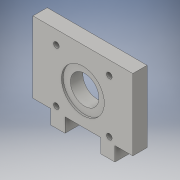
# Autodesk Inventor part: Motor Bracket
Saved by Autodesk Inventor 2016 (Build 200138000, 138)
## iProperties
Created: 2016-04-25
Part Number: Motor Bracket
Material: Generic
Document SubType Name: Modeling
Designer: rubenjm
Density: 1 g/cm^3
Appearance: Default
Author: rubenjm
Autodesk Inventor part; units mm, degrees
ref_plane "YZ Plane" through (0, 0, 0) normal (1, 0, 0) x (0, 1, 0)
ref_plane "XZ Plane" through (0, 0, 0) normal (0, 1, 0) x (-1, 0, 0)
ref_plane "XY Plane" through (0, 0, 0) normal (0, 0, 1) x (1, 0, 0)
sketch "Sketch1" plane through (0, 0, 0) normal (0, 0, 1) x (1, 0, 0)
  line L0 (0, 0) -> (15.875, 0)
  line L1 (88.9, 0) -> (88.9, 63.5)
  line L2 (88.9, 63.5) -> (0, 63.5)
  line L3 (0, 63.5) -> (0, 0)
  line L4 (44.45, 0) -> (60.325, 0) construction
  line L5 (44.45, 0) -> (60.325, 0) construction
  line L6 (73.025, 0) -> (73.025, -12.7)
  line L7 (73.025, -12.7) -> (60.325, -12.7)
  line L8 (60.325, -12.7) -> (60.325, 0)
  line L9 (73.025, 0) -> (88.9, 0)
  line L10 (44.45, 0) -> (44.45, 63.5) construction
  line L11 (44.45, 0) -> (28.575, 0) construction
  line L12 (44.45, 0) -> (28.575, 0) construction
  line L13 (15.875, 0) -> (15.875, -12.7)
  line L14 (15.875, -12.7) -> (28.575, -12.7)
  line L15 (28.575, -12.7) -> (28.575, 0)
  line L16 (28.575, 0) -> (60.325, 0)
  dimension "d10" = 88.9
  dimension "d11" = 63.5
  dimension "d12" = 15.875
  dimension "d13" = 0
  dimension "d14" = 12.7
  dimension "d15" = 12.7
  constraints: 34 end point, 5 parallel, 5 symmetric about line, 4 collinear, 4 horizontal, 3 perpendicular, 1 midpoint
  measures "d10" distance of L2.end L1.end
  measures "d11" distance of L1.end L1.start
  measures "d12" distance of L4.start L4.end
  measures "d13" distance between parallel lines of L4 L5
  measures "d14" distance of L6.end L7.end
  measures "d15" distance of L6.start L6.end
extrude "Extrusion1" add sketch "Sketch1" along normal blind 12.7
sketch "Sketch2" plane through (0, 0, 12.7) normal (0, 0, 1) x (1, 0, 0)
  line L0 (72.65, -0.26) -> (16.25, -0.26) construction
  line L1 (16.25, -0.26) -> (16.25, 56.14) construction
  line L2 (16.25, 56.14) -> (72.65, 56.14) construction
  line L3 (72.65, 56.14) -> (72.65, -0.26) construction
  line L4 (16.25, -0.26) -> (72.65, 56.14) construction
  line L5 (68.02, 4.37) -> (20.88, 4.37) construction
  line L6 (20.88, 4.37) -> (20.88, 51.51) construction
  line L7 (20.88, 51.51) -> (68.02, 51.51) construction
  line L8 (68.02, 51.51) -> (68.02, 4.37) construction
  line L9 (68.02, 4.37) -> (20.88, 51.51) construction
  line L10 (20.88, 4.37) -> (68.02, 51.51) construction
  circle A0 centre (20.8494, 4.3394) radius 2.5
  circle A1 centre (20.88, 51.51) radius 2.5
  circle A2 centre (68.02, 51.51) radius 2.5
  circle A3 centre (68.02, 4.37) radius 2.5
  line L11 (28.575, 0) -> (60.325, 0) construction
  line L12 (44.45, 0) -> (44.45, 27.94) construction
  line L13 (44.45, 0) -> (72.39, 0) construction
  point P0 (0, 0)
  point P1 (44.45, 27.94)
  dimension "d18" = 47.14
  dimension "d19" = 47.14
  dimension "d20" = 5
  dimension "d21" = 5
  dimension "d22" = 5
  dimension "d23" = 5
  dimension "d24" = 27.94
  dimension "d25" = 90
  constraints: 26 end point, 4 centre point, 4 midpoint, 4 parallel, 3 coincident, 3 horizontal, 3 perpendicular, 1 point on line, 1 vertical
  measures "d18" distance of L6.end L7.end
  measures "d19" distance of L5.end L6.end
  measures "d20" diameter of A0
  measures "d21" diameter of A1
  measures "d22" diameter of A2
  measures "d23" diameter of A3
  measures "d24" distance of L12.start L12.end
  measures "d25" angle of L13 L12
extrude "Extrusion2" cut sketch "Sketch2" against normal through all
sketch "Sketch3" plane through (0, 0, 12.7) normal (0, 0, 1) x (1, 0, 0)
  circle A0 centre (44.45, 27.94) radius 19.05
  line L0 (28.575, 0) -> (60.325, 0) construction
  line L1 (44.45, 0) -> (44.45, 27.94) construction
  point P0 (0, 0)
  dimension "d28" = 38.1
  dimension "d29" = 27.94
  constraints: 2 end point, 1 centre point, 1 midpoint, 1 vertical
  measures "d28" diameter of A0
  measures "d29" distance of L1.start L1.end
extrude "Extrusion3" cut sketch "Sketch3" against normal blind 1.6
sketch "Sketch4" plane through (44.45, 27.94, 11.1) normal (0, 0, 1) x (1, 0, 0)
  circle A0 centre (0, 0) radius 12.7
  point P0 (-44.45, -27.94)
  dimension "d32" = 25.4
  constraints: 1 centre point
  measures "d32" diameter of A0
extrude "Extrusion4" cut sketch "Sketch4" against normal through all
body "Solid1"
